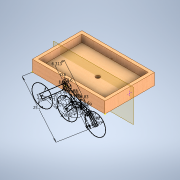
# Autodesk Inventor part: base
Saved by Autodesk Inventor 2020 (Build 240168000, 168)
## iProperties
Created: 2020-05-18
Part Number: base
Material: Wood (Cherry)
Document SubType Name: Modeling
Designer: Manish
Density: 0.63 g/cm^3
Appearance: Cherry - Natural Low Gloss
Author: Manish
Autodesk Inventor part; units mm, degrees
ref_plane "YZ Plane" through (0, 0, 0) normal (1, 0, 0) x (0, 1, 0)
ref_plane "XZ Plane" through (0, 0, 0) normal (0, 1, 0) x (-1, 0, 0)
ref_plane "XY Plane" through (0, 0, 0) normal (0, 0, 1) x (1, 0, 0)
sketch "Sketch3" plane through (0, 0, 0) normal (1, 0, 0) x (0, 1, 0)
  line L0 (0, 0) -> (55, 0)
  line L1 (55, 0) -> (55, -242)
  line L2 (55, -242) -> (0, -242)
  line L3 (0, -242) -> (0, 0)
  dimension "d4" = 55
  dimension "d5" = 242
  constraints: 8 end point, 2 parallel, 1 horizontal, 1 perpendicular
  measures "d4" distance of L1.end L2.end
  measures "d5" distance of L0.end L1.end
extrude "Extrusion3" add sketch "Sketch3" along normal blind 355
sketch "Sketch7" plane through (0, 55, 0) normal (0, 1, 0) x (1, 0, 0)
  circle A0 centre (200, 120) radius 10
  point P0 (0, 0)
  dimension "d20" = 20
  constraints: 1 centre point
  measures "d20" diameter of A0
extrude "Extrusion7" cut sketch "Sketch7" against normal through all
sketch "Sketch8" plane through (0, 55, 0) normal (0, 1, 0) x (1, 0, 0)
  line L0 (15, 15) -> (340, 15)
  line L1 (340, 15) -> (340, 227)
  line L2 (340, 227) -> (15, 227)
  line L3 (15, 227) -> (15, 15)
  line L4 (355, 242) -> (355, 0) projected
  line L5 (0, 242) -> (355, 242) projected
  point P0 (0, 0)
  dimension "d23" = 15
  dimension "d24" = 15
  constraints: 8 end point, 2 parallel, 1 horizontal, 1 perpendicular
  measures "d23" distance between parallel lines of L1 L4
  measures "d24" distance between parallel lines of L2 L5
extrude "Extrusion8" cut sketch "Sketch8" against normal blind 35
sketch "Sketch9" plane through (0, 0, 0) normal (0, 0, 1) x (1, 0, 0)
  circle A0 centre (161.4027, 23.0942) radius 3
  point P0 (0, 0)
  dimension "d27" = 6
  constraints: 1 centre point, 1 coincident
  measures "d27" diameter of A0
extrude "Extrusion9" cut sketch "Sketch9" against normal through all
sketch "Sketch10" plane through (0, 0, 0) normal (0, 0, 1) x (1, 0, 0)
  circle A0 centre (161.4027, 23.0942) radius 3 projected
  line L0 (161.4027, 23.0942) -> (154.8421, 30.6413)
  line L1 (154.8421, 30.6413) -> (167.9633, 15.5471)
  line L2 (159.3568, 8.0655) -> (47.2098, -89.4224)
  line L3 (47.2098, -89.4224) -> (34.0886, -74.3282)
  line L4 (34.0886, -74.3282) -> (157.0784, 32.5853)
  line L5 (167.9633, 15.5471) -> (175.5104, 22.1077)
  line L6 (175.5104, 22.1077) -> (162.3892, 37.2019)
  line L7 (162.3892, 37.2019) -> (154.8421, 30.6413)
  line L8 (161.4027, 23.0942) -> (168.0923, 30.6413)
  line L9 (168.0923, 30.6413) -> (154.826, 15.6744)
  line L10 (166.3278, 8.7133) -> (242.6544, -36.0367)
  line L11 (252.77, -18.7834) -> (164.0495, 33.233)
  line L12 (154.826, 15.6744) -> (147.3426, 22.3075)
  line L13 (147.3426, 22.3075) -> (160.6088, 37.2744)
  line L14 (165.473, 32.9629) -> (168.0923, 30.6413)
  circle A1 centre (236.8486, -22.4261) radius 3
  arc A2 (165.473, 32.9629) -> (157.5568, 33.0011) centre (161.4931, 28.4728) ccw
  arc A3 (166.8279, 8.3855) -> (159.3568, 8.0655) centre (163.2931, 3.5373) ccw
  line L15 (236.8486, -22.4261) -> (193.7959, -35.5206)
  line L16 (193.7959, -35.5206) -> (161.7278, -73.8826)
  line L17 (236.8486, -22.4261) -> (280.0214, -35.1189)
  line L18 (280.0214, -35.1189) -> (312.2613, -73.3366)
  line L19 (236.8486, -22.4261) -> (233.9392, -12.8604)
  line L20 (236.8486, -22.4261) -> (239.7585, -31.9934)
  line L21 (193.7959, -35.5206) -> (190.6756, -25.2616)
  line L22 (193.7959, -35.5206) -> (196.7058, -45.0879)
  line L23 (235.2146, -12.4948) -> (196.0322, -23.7261)
  line L24 (206.7188, -42.0424) -> (235.1804, -33.3858)
  line L25 (193.7959, -35.5206) -> (203.8613, -43.9346)
  line L26 (193.7959, -35.5206) -> (186.1235, -29.107)
  line L27 (203.8613, -43.9346) -> (171.7932, -82.2966)
  line L28 (171.7932, -82.2966) -> (156.4485, -69.4693)
  line L29 (156.4485, -69.4693) -> (193.0821, -25.6457)
  line L30 (236.8486, -22.4261) -> (237.4753, -12.4458)
  line L31 (236.8486, -22.4261) -> (234.028, -32.0201)
  line L32 (280.0214, -35.1189) -> (282.842, -25.525)
  line L33 (282.842, -25.525) -> (277.2008, -44.7129)
  line L34 (238.6187, -33.3698) -> (272.5858, -43.3561)
  line L35 (283.9958, -25.8642) -> (238.5602, -12.5061)
  line L36 (280.0214, -35.1189) -> (287.6649, -28.671)
  line L37 (280.0214, -35.1189) -> (272.3779, -41.5669)
  line L38 (312.2613, -73.3366) -> (319.9048, -66.8886)
  line L39 (319.9048, -66.8886) -> (304.6177, -79.7846)
  line L40 (304.6177, -79.7846) -> (275.4795, -45.2437)
  line L41 (319.9048, -66.8886) -> (286.8895, -27.7518)
  arc A4 (196.0322, -23.7261) -> (193.0821, -25.6457) centre (197.6855, -29.4939) ccw
  arc A5 (206.7188, -42.0424) -> (203.8613, -43.9346) centre (208.4647, -47.7828) ccw
  arc A6 (236.3138, -12.2881) -> (233.3029, -13.4364) centre (236.8679, -18.2625) ccw
  arc A7 (238.6187, -33.3698) -> (235.1804, -33.3858) centre (236.9264, -39.1262) ccw
  arc A8 (286.8895, -27.7518) -> (283.9958, -25.8642) centre (282.3034, -31.6205) ccw
  arc A9 (275.4795, -45.2437) -> (272.5858, -43.3561) centre (270.8934, -49.1125) ccw
  arc A10 (164.0495, 33.233) -> (157.0784, 32.5853) centre (161.0148, 28.057) ccw
  arc A11 (166.3278, 8.7133) -> (159.3568, 8.0655) centre (163.2931, 3.5373) ccw
  arc A12 (238.5602, -12.5061) -> (235.2146, -12.4948) centre (236.8679, -18.2625) ccw
  line L42 (242.6544, -36.0367) -> (252.77, -18.7834)
  circle A13 centre (47.2098, -76.1722) radius 50
  circle A14 centre (306.8219, -66.8886) radius 50
  circle A15 centre (169.4822, -69.4693) radius 50
  point P0 (0, 0)
  point P1 (188.5165, -31.1074)
  dimension "d34" = 20
  dimension "d35" = 160
  dimension "d36" = 20
  dimension "d38" = 10
  dimension "d39" = 20
  dimension "d42" = 10
  dimension "d43" = 20
  dimension "d46" = 6
  dimension "d47" = 6
  dimension "d48" = 6
  dimension "d53" = 45
  dimension "d55" = 10
  dimension "d56" = 20
  dimension "d57" = 50
  dimension "d58" = 10
  dimension "d59" = 10
  dimension "d60" = 10
  dimension "d61" = 20
  dimension "d62" = 10
  dimension "d63" = 10
  dimension "d64" = 10
  dimension "d65" = 20
  dimension "d66" = 6
  dimension "d67" = 6
  dimension "d68" = 50
  dimension "d69" = 10
  dimension "d70" = 33.466
  dimension "d72" = 66.767
  dimension "d73" = 24.156
  dimension "d74" = 99.956
  dimension "d75" = 359.15
  dimension "d76" = 170.9804
  dimension "d77" = 63.131
  dimension "d78" = 54.5499
  dimension "d79" = 10
  dimension "d80" = 257.4003
  dimension "d83" = 6
  dimension "d84" = 108.617
  dimension "d85" = 102.79
  dimension "d86" = 64.83
  dimension "d87" = 154.83
  dimension "d88" = 20
  dimension "d89" = 100
  dimension "d90" = 78.1505
  dimension "d91" = 10.0851
  dimension "d92" = 10.0851
  dimension "d93" = 9.7519
  dimension "d94" = 9.5755
  dimension "d95" = 7.6246
  dimension "d96" = 31.5191
  dimension "d97" = 31.5191
  dimension "d98" = 9.8104
  dimension "d99" = 100
  dimension "d100" = 100
  dimension "d101" = 100
  dimension "d102" = 22.9203
  dimension "d103" = 64.1346
  dimension "d104" = 15.4047
  dimension "d105" = 105.0537
  dimension "d106" = 13.7623
  constraints: 86 end point, 24 point on line, 22 point on circle, 20 tangent, 18 perpendicular, 15 centre point, 7 parallel, 6 equal radius, 3 equal length, 2 coincident
  measures "d34" distance of L0.end L1.end
  measures "d35" distance of L1.end L2.end
  measures "d36" distance of L2.end L3.end
  measures "d38" distance of L1.end L5.end
  measures "d39" distance of L9.start L9.end
  measures "d42" distance of L9.end L12.end
  measures "d43" distance of L12.end L13.end
  measures "d46" diameter of A1
  measures "d47" radius of A2
  measures "d48" radius of A3
  measures "d53" distance between parallel lines of L20 L22
  measures "d55" distance of L15.end L26.end
  measures "d56" distance of L27.end L28.end
  measures "d57" distance between parallel lines of L26 L28
  measures "d58" distance of L30.start L30.end
  measures "d59" distance of L15.start L31.end
  measures "d60" distance of L17.end L32.end
  measures "d61" distance of L32.end L33.end
  measures "d62" distance of L17.end L36.end
  measures "d63" distance of L17.end L37.end
  measures "d64" distance of L18.end L38.end
  measures "d65" distance of L38.end L39.end
  measures "d66" radius of A4
  measures "d67" radius of A6
  measures "d68" distance between parallel lines of L39 L37
  measures "d69" distance between parallel lines of L24 L15
  measures "d70" angle of L32 L39
  measures "d72" angle of L39 L20
  measures "d73" angle of L23 L39
  measures "d74" angle of L39 L25
  measures "d76" distance from line of A0.centre L39
  measures "d77" distance from line of A0.centre L41
  measures "d78" distance from line of A0.centre L23
  measures "d79" distance from line of A0.centre L5
  measures "d80" distance from line of point (0, 0) L39
  measures "d83" radius of A10
  measures "d84" angle of L10 L2
  measures "d85" angle of L17 L30
  measures "d86" angle of L8 L17
  measures "d87" angle of L14 L17
  measures "d88" distance between parallel lines of L11 L10
  measures "d89" distance from line of A0.centre L42
  measures "d90" distance from line of A0.centre L30
  measures "d91" distance from line of A0.centre L11
  measures "d92" distance from line of A0.centre L14
  measures "d93" distance from line of L30.end L17
  measures "d94" distance from line of A6.start L17
  measures "d95" distance from line of A6.end L17
  measures "d96" distance from line of L8.end L17
  measures "d97" distance from line of L14.end L17
  measures "d98" distance from line of A3.start L17
  measures "d99" diameter of A13
  measures "d100" diameter of A14
  measures "d101" diameter of A15
  measures "d102" distance from line of A14.centre L17
  measures "d103" distance from line of A15.centre L17
  measures "d104" distance from line of A15.centre L24
  measures "d105" distance from line of A13.centre L17
  measures "d106" distance from line of A13.centre L24
ref_plane "Work Plane1" through (0, 0, -121) normal (0, 0, 1) x (1, 0, 0)
sketch "Sketch13" plane through (355, 0, 0) normal (1, 0, 0) x (0, 0, -1)
  point P0 (0, 0)
  point P1 (121, 27.5)
  point P2 (121, 27.5)
  constraints: 1 coincident
sketch "Sketch14" plane through (0, 0, 0) normal (-1, 0, 0) x (0, 0, 1)
  point P0 (0, 0)
  point P1 (-121, 27.5)
body "Solid2"
